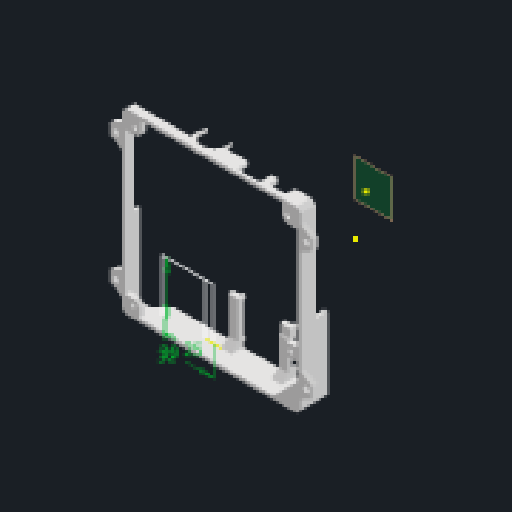
# Autodesk Inventor part: Buttom_part
Saved by Autodesk Inventor 2026.2 (Build 302298000, 298)
## iProperties
Created: 2026-04-25
Part Number: Buttom_part
Material: Generic
Document SubType Name: Modeling
Designer: Malthe Sennels
Density: 1 g/cm^3
Appearance: Default
Author: Malthe Sennels
Autodesk Inventor part; units mm, degrees
ref_plane "YZ Plane" through (0, 0, 0) normal (1, 0, 0) x (0, 1, 0)
ref_plane "XZ Plane" through (0, 0, 0) normal (0, 1, 0) x (-1, 0, 0)
ref_plane "XY Plane" through (0, 0, 0) normal (0, 0, 1) x (1, 0, 0)
sketch "Sketch1" plane through (0, 0, 0) normal (0, 0, 1) x (1, 0, 0)
  line L0 (-32, -107.75) -> (-32, -22.5) construction
  line L1 (-33, -21.5) -> (-131, -21.5) construction
  line L2 (-32, -22.5) -> (-33, -21.5) construction
  line L3 (-45.75, -121.5) -> (-32, -107.75) construction
  line L4 (-131, -121.5) -> (-45.75, -121.5) construction
  line L5 (-132, -120.5) -> (-131, -121.5) construction
  line L6 (-132, -22.5) -> (-132, -120.5) construction
  line L7 (-131, -21.5) -> (-132, -22.5) projected
  line L8 (-31.6, -22.3343) -> (-31.6, -107.9157)
  line L9 (-31.6, -107.9157) -> (-45.5843, -121.9)
  line L10 (-45.5843, -121.9) -> (-131.1657, -121.9)
  line L11 (-131.1657, -121.9) -> (-132.4, -120.6657)
  line L12 (-132.4, -120.6657) -> (-132.4, -22.3343)
  line L13 (-132.4, -22.3343) -> (-131.1657, -21.1)
  line L14 (-131.1657, -21.1) -> (-32.8343, -21.1)
  line L15 (-32.8343, -21.1) -> (-31.6, -22.3343)
  circle A0 centre (-37, -26.5) radius 1.25 projected
  circle A1 centre (-37, -26.5) radius 3.75
  line L16 (-40.75, -26.5) -> (-40.75, -21.1)
  line L17 (-37, -30.25) -> (-31.6, -30.25)
  circle A2 centre (-126.8952, -26.4793) radius 1.25 projected
  circle A3 centre (-126.8952, -26.4793) radius 3.75
  line L18 (-123.1452, -26.4793) -> (-123.1452, -21.1)
  line L19 (-126.8952, -30.2293) -> (-132.4, -30.2293)
  circle A4 centre (-127.9242, -117.4242) radius 1.25 projected
  circle A5 centre (-127.9242, -117.4242) radius 3.75
  line L20 (-124.1742, -117.4242) -> (-124.1742, -121.9)
  line L21 (-127.9242, -113.6742) -> (-132.4, -113.6742)
  circle A6 centre (-35.375, -94.25) radius 1.25 projected
  circle A7 centre (-35.375, -94.25) radius 3.75
  line L22 (-35.375, -98) -> (-31.6, -98)
  line L23 (-35.375, -90.5) -> (-31.6, -90.5)
  line L24 (-29.6, -108.7441) -> (-29.6, -21.5059)
  line L25 (-29.6, -21.5059) -> (-32.0059, -19.1)
  line L26 (-32.0059, -19.1) -> (-131.9941, -19.1)
  line L27 (-131.9941, -19.1) -> (-134.4, -21.5059)
  line L28 (-134.4, -21.5059) -> (-134.4, -121.4941)
  line L29 (-134.4, -121.4941) -> (-131.9941, -123.9)
  line L30 (-131.9941, -123.9) -> (-44.7559, -123.9)
  line L31 (-44.7559, -123.9) -> (-29.6, -108.7441)
  line L32 (-29.6, -108.7441) -> (-29.6, -121.4941)
  line L33 (-32.0059, -123.9) -> (-44.7559, -123.9)
  line L34 (-29.6, -121.4941) -> (-32.0059, -123.9)
  point P0 (0, 0)
  point P1 (-29.6, -123.9)
  dimension "d0" = 0.4
  dimension "d1" = 7.5
  dimension "d2" = 7.5
  dimension "d3" = 7.5
  dimension "d4" = 7.5
  dimension "d5" = 2
  dimension "d26" = 2.4059
  dimension "d27" = 2.4059
  dimension "d28" = 2.4059
  constraints: 54 end point, 11 point on line, 8 perpendicular, 8 point on circle, 8 tangent, 4 centre point, 4 coincident, 1 vertical, 14 other
  measures "d0" distance between parallel lines of L0 L8
  measures "d1" diameter of A1
  measures "d2" diameter of A3
  measures "d3" diameter of A5
  measures "d4" diameter of A7
  measures "d5" distance between parallel lines of L8 L24
  measures "d26" horizontal distance of L28.end L29.end
  measures "d27" distance of L32.end point (-29.6, -123.9)
  measures "d28" distance of L33.start point (-29.6, -123.9)
extrude "Extrusion1" add sketch "Sketch1" along normal blind 3 contours L8 L17 A1 L16 L14 L15 | L8 L22 A7 L23 | A1 | A7 | L18 A3 L19 L12 L13 L14 | A3 | L10 L11 L12 L21 A5 L20 | A5 | L31 L30 L29 L28 L27 L26 L25 L24 | L32 L34 L33 L31
sketch "Sketch3" plane through (0, 0, 0) normal (0, 0, -1) x (-1, 0, 0)
  line L0 (29.6, -21.5059) -> (32.0059, -19.1) projected
  line L1 (134.4, -121.4941) -> (131.9941, -123.9) projected
  line L2 (134.4, -21.5059) -> (134.4, -121.4941) projected
  line L3 (131.9941, -19.1) -> (134.4, -21.5059) projected
  line L4 (32.0059, -19.1) -> (131.9941, -19.1) projected
  circle A0 centre (35.375, -94.25) radius 1.25 projected
  circle A1 centre (127.9242, -117.4242) radius 1.25 projected
  circle A2 centre (37, -26.5) radius 1.25 projected
  circle A3 centre (126.8952, -26.4793) radius 1.25 projected
  arc A4 (123.1452, -26.4793) -> (126.8952, -30.2293) centre (126.8952, -26.4793) ccw projected
  line L5 (132.4, -30.2293) -> (126.8952, -30.2293) projected
  line L6 (132.4, -113.6742) -> (132.4, -30.2293) projected
  line L7 (127.9242, -113.6742) -> (132.4, -113.6742) projected
  arc A5 (127.9242, -113.6742) -> (124.1742, -117.4242) centre (127.9242, -117.4242) ccw projected
  line L8 (124.1742, -121.9) -> (124.1742, -117.4242) projected
  line L9 (45.5843, -121.9) -> (124.1742, -121.9) projected
  line L10 (31.6, -107.9157) -> (45.5843, -121.9) projected
  line L11 (31.6, -98) -> (31.6, -107.9157) projected
  line L12 (35.375, -98) -> (31.6, -98) projected
  arc A6 (35.375, -98) -> (35.375, -90.5) centre (35.375, -94.25) ccw projected
  line L13 (31.6, -90.5) -> (35.375, -90.5) projected
  line L14 (31.6, -30.25) -> (31.6, -90.5) projected
  line L15 (37, -30.25) -> (31.6, -30.25) projected
  arc A7 (37, -30.25) -> (40.75, -26.5) centre (37, -26.5) ccw projected
  line L16 (40.75, -21.1) -> (40.75, -26.5) projected
  line L17 (123.1452, -21.1) -> (40.75, -21.1) projected
  line L18 (123.1452, -26.4793) -> (123.1452, -21.1) projected
  line L19 (31.6, -22.3343) -> (32.8343, -21.1)
  line L20 (32.8343, -21.1) -> (131.1657, -21.1)
  line L21 (131.1657, -21.1) -> (132.4, -22.3343)
  line L22 (132.4, -22.3343) -> (132.4, -120.6657)
  line L23 (132.4, -120.6657) -> (131.1657, -121.9)
  line L24 (131.1657, -121.9) -> (45.5843, -121.9)
  line L25 (45.5843, -121.9) -> (31.6, -107.9157)
  line L26 (31.6, -107.9157) -> (31.6, -22.3343)
  line L27 (29.6, -121.4941) -> (29.6, -21.5059) projected
  line L28 (32.0059, -123.9) -> (29.6, -121.4941) projected
  line L29 (131.9941, -123.9) -> (32.0059, -123.9) projected
  point P0 (0, 0)
  point P1 (132.4, -41.5929)
  constraints: 16 end point, 4 other
extrude "Extrusion2" add sketch "Sketch3" along normal blind 6 contours L0 L4 L3 L2 L1 L29 L28 L27
sketch "Sketch4" plane through (-131.9941, -19.1, 3) normal (0, 1, 0) x (1, 0, 0)
  line L0 (65.2616, 3) -> (65.2616, 4.5558) projected
  line L1 (74.5016, 3) -> (74.5016, 4.5558) projected
  line L2 (98.9941, 3) -> (0.9941, 3) projected
  line L3 (99.1598, 9) -> (0.8284, 9) projected
  line L4 (63.2616, 8) -> (63.2616, 3)
  line L5 (64.2616, 2) -> (75.5016, 2)
  line L6 (76.5016, 3) -> (76.5016, 8)
  arc A0 (63.2616, 3) -> (64.2616, 2) centre (64.2616, 3) ccw
  arc A1 (75.5016, 2) -> (76.5016, 3) centre (75.5016, 3) ccw
  line L7 (62.2616, 9) -> (61.3217, 9)
  line L8 (77.5016, 9) -> (78.7059, 9)
  line L9 (63.2616, 9) -> (76.5016, 9)
  arc A2 (63.2616, 8) -> (62.2616, 9) centre (62.2616, 8) ccw
  arc A3 (77.5016, 9) -> (76.5016, 8) centre (77.5016, 8) ccw
  line L10 (87.1737, 4.5558) -> (88.7737, 4.5558) projected
  line L11 (82.0937, 4.5558) -> (83.6937, 4.5558) projected
  line L12 (80.5937, 8) -> (80.5937, 4.5558)
  line L13 (81.5937, 3.5558) -> (89.2737, 3.5558)
  line L14 (90.2737, 4.5558) -> (90.2737, 8)
  arc A4 (80.5937, 4.5558) -> (81.5937, 3.5558) centre (81.5937, 4.5558) ccw
  arc A5 (89.2737, 3.5558) -> (90.2737, 4.5558) centre (89.2737, 4.5558) ccw
  line L15 (77.5016, 9) -> (79.5937, 9)
  arc A6 (80.5937, 8) -> (79.5937, 9) centre (79.5937, 8) ccw
  line L16 (102.3941, 9) -> (102.3941, 0) projected
  line L17 (91.2737, 9) -> (102.3941, 9)
  arc A7 (91.2737, 9) -> (90.2737, 8) centre (91.2737, 8) ccw
  point P0 (131.9941, 3)
  point P1 (80.5937, 9)
  point P2 (90.2737, 9)
  dimension "d11" = 2
  dimension "d12" = 2
  dimension "d13" = 1
  dimension "d14" = 1
  dimension "d15" = 1
  dimension "d32" = 1.5
  dimension "d33" = 1.5
  dimension "d34" = 1
  dimension "d35" = 1
  dimension "d36" = 1
  dimension "d37" = 1
  constraints: 22 end point, 16 point on circle, 16 tangent, 14 point on line, 8 centre point, 4 perpendicular, 3 equal radius, 2 horizontal, 2 vertical, 1 collinear
  measures "d11" distance between parallel lines of L6 L1
  measures "d12" distance between parallel lines of L4 L0
  measures "d13" distance between parallel lines of L2 L5
  measures "d14" radius of A0
  measures "d15" radius of A2
  measures "d32" distance from line of L12 L11.start
  measures "d33" distance from line of L14 L10.end
  measures "d34" distance between parallel lines of L11 L13
  measures "d35" radius of A4
  measures "d36" radius of A6
  measures "d37" radius of A7
extrude "Extrusion3" cut sketch "Sketch4" against normal up to surface (2 mm away)
sketch "Sketch5" plane through (0, 0, 3) normal (0, 0, 1) x (1, 0, 0)
  circle A0 centre (-26.1, -34.1) radius 1.75
  line L0 (-29.6, -108.7441) -> (-29.6, -21.5059) projected
  line L1 (-29.6, -27.0585) -> (-22.6, -31.1)
  line L2 (-22.6, -31.1) -> (-22.6, -37.1)
  line L3 (-22.6, -37.1) -> (-29.6, -41.1415)
  line L4 (-22.6, -34.1) -> (-29.6, -34.1) construction
  line L5 (-32.0059, -19.1) -> (-131.9941, -19.1) projected
  line L6 (-29.6, -21.5059) -> (-29.6, -121.4941)
  line L7 (-29.6, -71.5) -> (-134.4, -71.5)
  line L8 (-134.4, -21.5059) -> (-134.4, -121.4941) projected
  circle A1 centre (-26.1, -108.9) radius 1.75
  line L9 (-29.6, -115.9415) -> (-22.6, -111.9)
  line L10 (-22.6, -111.9) -> (-22.6, -105.9)
  line L11 (-22.6, -105.9) -> (-29.6, -101.8585)
  line L12 (-22.6, -108.9) -> (-29.6, -108.9) construction
  line L13 (-82, -19.1) -> (-82, -123.9)
  line L14 (-131.9941, -123.9) -> (-32.0059, -123.9) projected
  circle A2 centre (-137.9, -34.1) radius 1.75
  line L15 (-134.4, -27.0585) -> (-141.4, -31.1)
  line L16 (-141.4, -31.1) -> (-141.4, -37.1)
  line L17 (-141.4, -37.1) -> (-134.4, -41.1415)
  line L18 (-141.4, -34.1) -> (-134.4, -34.1) construction
  line L19 (-134.4, -115.9415) -> (-141.4, -111.9)
  line L20 (-141.4, -108.9) -> (-134.4, -108.9) construction
  circle A3 centre (-137.9, -108.9) radius 1.75
  line L21 (-141.4, -105.9) -> (-134.4, -101.8585)
  line L22 (-141.4, -111.9) -> (-141.4, -105.9)
  point P0 (0, 0)
  point P1 (-134.4, -108.7441)
  dimension "d19" = 120
  dimension "d20" = 120
  dimension "d21" = 3.5
  dimension "d22" = 3.5
  dimension "d23" = 7
  dimension "d24" = 3
  dimension "d25" = 15
  constraints: 38 end point, 22 symmetric about line, 9 midpoint, 4 centre point, 3 point on line, 1 parallel, 1 perpendicular, 3 other
  measures "d19" angle of L2 L3
  measures "d20" angle of L2 L1
  measures "d21" distance from line of L0 A0.centre
  measures "d22" diameter of A0
  measures "d23" distance between parallel lines of L0 L2
  measures "d24" distance from line of L1.end L4
  measures "d25" distance between parallel lines of L5 L4
extrude "Extrusion4" add sketch "Sketch5" against normal blind 3
sketch "Sketch6" plane through (0, 0, -6) normal (0, 0, -1) x (-1, 0, 0)
  point P0 (0, 0)
sketch "Sketch7" plane through (-131.9941, -19.1, 3) normal (0, 1, 0) x (1, 0, 0)
  circle A0 centre (40.9941, 10.95) radius 3.9 projected
  circle A1 centre (40.9941, 10.95) radius 2.9
  line L0 (0, 9) -> (62.2616, 9) projected
  line L1 (49.2757, 9) -> (48.3941, 14)
  line L2 (48.3941, 14) -> (43.8941, 14)
  line L3 (43.8941, 14) -> (43.8941, 10.95)
  line L4 (40.9941, 7.05) -> (40.9941, 14.85)
  line L5 (32.7125, 9) -> (33.5941, 14)
  line L6 (33.5941, 14) -> (38.0941, 14)
  line L7 (38.0941, 14) -> (38.0941, 10.95)
  point P0 (131.9941, 3)
  point P1 (43.1406, 9)
  point P2 (32.7125, 9)
  point P3 (38.8476, 9)
  dimension "d38" = 5.8
  dimension "d39" = 80
  dimension "d40" = 5
  dimension "d41" = 4.5
  constraints: 14 end point, 4 symmetric about line, 3 vertical, 2 point on circle, 1 coincident, 1 parallel, 1 perpendicular, 1 point on line, 3 other
  measures "d39" angle of L0 L1
  measures "d40" distance between parallel lines of L0 L2
  measures "d41" distance of L2.end L1.end
extrude "Extrusion5" add sketch "Sketch7" against normal up to surface (2 mm away) contours A0 L0 A1 L3 | A0 L3 L2 L1 L0 | L7 A1 L0 A0 | A0 L0 L5 L6 L7
sketch "Sketch8" plane through (-131.9941, -19.1, 3) normal (0, 1, 0) x (1, 0, 0)
  arc A0 (43.1406, 9) -> (43.8941, 10.95) centre (40.9941, 10.95) ccw projected
  circle A1 centre (40.9941, 10.95) radius 2.9
  point P0 (131.9941, 3)
  point P1 (43.1406, 9)
  constraints: 1 coincident, 3 other
extrude "Extrusion6" cut sketch "Sketch8" against normal up to surface (2 mm away)
sketch "Sketch9" plane through (0, 0, -6) normal (0, 0, -1) x (-1, 0, 0)
  line L0 (94.6, -132.1582) -> (23.2926, -132.1582)
  line L1 (23.2926, -132.1582) -> (23.2926, -78.9)
  line L2 (23.2926, -78.9) -> (94.6, -78.9)
  line L3 (94.6, -78.9) -> (94.6, -132.1582)
  line L4 (99.2816, -19.1) -> (99.2816, -21.1) projected
  line L5 (99.2816, -21.1) -> (131.1657, -21.1) projected
  line L6 (131.1657, -21.1) -> (132.4, -22.3343) projected
  line L7 (132.4, -22.3343) -> (132.4, -120.6657) projected
  line L8 (132.4, -120.6657) -> (131.1657, -121.9) projected
  line L9 (131.1657, -121.9) -> (45.5843, -121.9) projected
  line L10 (45.5843, -121.9) -> (31.6, -107.9157) projected
  line L11 (31.6, -107.9157) -> (31.6, -22.3343) projected
  line L12 (31.6, -22.3343) -> (32.8343, -21.1) projected
  line L13 (32.8343, -21.1) -> (40.7204, -21.1) projected
  line L14 (40.7204, -21.1) -> (40.7204, -19.1) projected
  line L15 (40.7204, -19.1) -> (32.0059, -19.1) projected
  line L16 (32.0059, -19.1) -> (29.6, -21.5059) projected
  line L17 (29.6, -21.5059) -> (29.6, -121.4941) projected
  line L18 (29.6, -121.4941) -> (32.0059, -123.9) projected
  line L19 (32.0059, -123.9) -> (131.9941, -123.9) projected
  line L20 (131.9941, -123.9) -> (134.4, -121.4941) projected
  line L21 (134.4, -121.4941) -> (134.4, -21.5059) projected
  line L22 (134.4, -21.5059) -> (131.9941, -19.1) projected
  line L23 (131.9941, -19.1) -> (99.2816, -19.1) projected
  line L24 (32.0059, -123.9) -> (131.9941, -123.9) projected
  line L25 (29.6, -21.5059) -> (29.6, -121.4941) projected
  point P0 (0, 0)
  point P1 (31.6, -78.9)
  point P2 (29.6, -78.9)
  point P3 (94.6, -123.9)
  point P4 (94.6, -121.9)
  dimension "d46" = 45
  dimension "d47" = 65
  constraints: 8 end point, 2 parallel, 1 horizontal, 1 perpendicular
  measures "d46" distance between parallel lines of L2 L24
  measures "d47" distance between parallel lines of L3 L25
extrude "Extrusion7" add sketch "Sketch9" along normal blind 7 contours L19 L18 L17 L2 L11 L10 L9 L3
sketch "Sketch10" plane through (0, 0, -13) normal (0, 0, -1) x (-1, 0, 0)
  line L0 (32.0059, -123.9) -> (94.6, -123.9) projected
  line L1 (54.6, -123.9) -> (48.6, -123.9)
  line L2 (48.6, -123.9) -> (48.6, -95.9)
  line L3 (48.6, -95.9) -> (54.6, -95.9)
  line L4 (54.6, -95.9) -> (54.6, -123.9)
  line L5 (85.08, -123.9) -> (79.08, -123.9)
  line L6 (79.08, -123.9) -> (79.08, -95.9)
  line L7 (79.08, -95.9) -> (85.08, -95.9)
  line L8 (85.08, -95.9) -> (85.08, -123.9)
  line L9 (82.08, -95.9) -> (82.08, -123.9)
  line L10 (51.6, -95.9) -> (51.6, -123.9)
  line L11 (29.6, -78.9) -> (29.6, -121.4941) projected
  point P0 (0, 0)
  dimension "d50" = 30.48
  dimension "d51" = 6
  dimension "d52" = 6
  dimension "d53" = 28
  dimension "d54" = 22
  constraints: 20 end point, 4 midpoint, 4 parallel, 3 point on line, 2 horizontal, 2 perpendicular
  measures "d50" distance between parallel lines of L10 L9
  measures "d51" distance between parallel lines of L2 L4
  measures "d52" distance between parallel lines of L8 L6
  measures "d53" distance between parallel lines of L0 L7
  measures "d54" distance between parallel lines of L11 L10
extrude "Extrusion8" add sketch "Sketch10" against normal blind 3
sketch "Sketch11" plane through (0, 0, -13) normal (0, 0, -1) x (-1, 0, 0)
  line L0 (79.08, -95.9) -> (85.08, -95.9) projected
  line L1 (82.08, -95.9) -> (82.08, -125.121) construction
  line L2 (54.6, -95.9) -> (48.6, -95.9) projected
  line L3 (51.6, -95.9) -> (51.6, -123.9) construction
  line L4 (32.0059, -123.9) -> (94.6, -123.9) projected
  circle A0 centre (82.08, -120.16) radius 1.4
  circle A1 centre (82.08, -98.9) radius 1.4
  line L5 (85.08, -95.9) -> (79.08, -95.9) projected
  line L6 (82.08, -120.16) -> (51.6, -120.16)
  line L7 (82.08, -98.9) -> (51.6, -98.9)
  circle A2 centre (51.6, -120.16) radius 1.4
  circle A3 centre (51.6, -98.9) radius 1.4
  point P0 (0, 0)
  dimension "d57" = 2.8
  dimension "d58" = 2.8
  dimension "d59" = 21.26
  dimension "d60" = 3
  dimension "d61" = 2.8
  dimension "d62" = 2.8
  constraints: 8 end point, 5 point on line, 4 centre point, 2 coincident, 2 midpoint, 2 perpendicular, 2 vertical
  measures "d57" diameter of A0
  measures "d58" diameter of A1
  measures "d59" distance of L7.start L6.start
  measures "d60" distance from line of L5 L7.start
  measures "d61" diameter of A2
  measures "d62" diameter of A3
extrude "Extrusion9" add sketch "Sketch11" along normal blind 3
sketch "Sketch12" plane through (-48.6, -121.9, -13) normal (1, 0, 0) x (0, 0, -1)
  line L0 (0, 20) -> (-2, 18)
  line L1 (-2, 18) -> (-2, 7)
  line L2 (-2, 7) -> (0, 5)
  line L3 (0, 0) -> (0, 26) projected
  line L4 (0, 0) -> (0, 26) projected
  line L5 (-7, -2) -> (0, -2) projected
  point P0 (-13, 121.9)
  point P1 (0, 13)
  point P2 (0, 20)
  dimension "d65" = 135
  dimension "d66" = 135
  dimension "d67" = 2
  dimension "d68" = 8
  dimension "d69" = 9
  constraints: 6 end point, 2 point on line, 1 midpoint, 1 parallel
  measures "d65" angle of L4 L0
  measures "d66" angle of L4 L2
  measures "d67" distance from line of point (0, 13) L1
  measures "d68" vertical distance of L3.end L0.end
  measures "d69" distance from line of L1.end L5
extrude "Extrusion10" cut sketch "Sketch12" against normal up to surface (6 mm away)
sketch "Sketch13" plane through (-48.6, -121.9, -10) normal (1, 0, 0) x (0, 0, -1)
  line L0 (3, 20) -> (1, 18) projected
  line L1 (1, 7) -> (3, 5) projected
  line L2 (1, 22.2426) -> (-1, 20.2426)
  line L3 (-1.1213, 4.8787) -> (0.8787, 2.8787)
  line L4 (-1, 20.2426) -> (-1, 0)
  line L5 (-4, 0) -> (3, 0) projected
  line L6 (3, 0) -> (3, 5) projected
  line L7 (0, 21.2426) -> (0, 0)
  point P0 (-10, 121.9)
  dimension "d72" = 3
  dimension "d73" = 3
  dimension "d74" = 4
  constraints: 8 end point, 3 point on line, 2 parallel, 2 perpendicular, 1 midpoint
  measures "d72" distance between parallel lines of L0 L2
  measures "d73" distance between parallel lines of L1 L3
  measures "d74" distance between parallel lines of L6 L4
extrude "Extrusion11" add sketch "Sketch13" against normal up to surface (6 mm away)
chamfer "Chamfer1" distance 4 angle 45 2 edges at (-82.08, -121.9, -10) (-51.6, -121.9, -9)
sketch "Sketch14" plane through (0, 0, -6) normal (0, 0, -1) x (-1, 0, 0)
  line L0 (94.6, -123.9) -> (131.9941, -123.9) projected
  line L1 (94.6, -123.9) -> (119.6, -123.9)
  line L2 (119.6, -123.9) -> (119.6, -91.9)
  line L3 (119.6, -91.9) -> (94.6, -91.9)
  line L4 (94.6, -91.9) -> (94.6, -123.9)
  line L5 (94.6, -121.9) -> (85.08, -121.9) projected
  line L6 (94.6, -91.9) -> (89.6, -91.9)
  line L7 (89.6, -91.9) -> (89.6, -121.9)
  line L8 (89.6, -121.9) -> (94.6, -121.9)
  line L9 (94.6, -121.9) -> (94.6, -91.9)
  point P0 (0, 0)
  dimension "d80" = 32
  dimension "d81" = 25
  dimension "d82" = 30
  constraints: 16 end point, 4 parallel, 2 horizontal, 2 perpendicular, 1 point on line
  measures "d80" distance between parallel lines of L0 L3
  measures "d81" distance between parallel lines of L4 L2
  measures "d82" distance between parallel lines of L2 L7
ref_plane "Work Plane1" through (0, 0, -10) normal (0, 0, -1) x (-1, 0, 0)
sketch "Sketch15" plane through (0, 0, -10) normal (0, 0, -1) x (-1, 0, 0)
  line L0 (94.6, -123.9) -> (94.6, -121.9) projected
  line L1 (94.6, -123.9) -> (119.6, -123.9) projected
  line L2 (119.6, -123.9) -> (119.6, -91.9) projected
  line L3 (119.6, -121.9) -> (94.6, -121.9)
  point P0 (0, 0)
  constraints: 2 end point, 1 horizontal, 1 point on line
extrude "Extrusion13" add sketch "Sketch15" along normal up to surface (3 mm away)
sketch "Sketch16" plane through (0, 0, -6) normal (0, 0, -1) x (-1, 0, 0)
  line L0 (145.0581, -74.1) -> (99.4, -74.1)
  line L1 (99.4, -74.1) -> (99.4, -16.8745)
  line L2 (99.4, -16.8745) -> (145.0581, -16.8745)
  line L3 (145.0581, -16.8745) -> (145.0581, -74.1)
  line L4 (94.6, -123.9) -> (131.9941, -123.9) projected
  line L5 (131.9941, -123.9) -> (134.4, -121.4941) projected
  line L6 (134.4, -121.4941) -> (134.4, -21.5059) projected
  line L7 (134.4, -21.5059) -> (131.9941, -19.1) projected
  line L8 (131.9941, -19.1) -> (99.2816, -19.1) projected
  line L9 (99.2816, -19.1) -> (99.2816, -21.1) projected
  line L10 (99.2816, -21.1) -> (131.1657, -21.1) projected
  line L11 (131.1657, -21.1) -> (132.4, -22.3343) projected
  line L12 (132.4, -22.3343) -> (132.4, -120.6657) projected
  line L13 (132.4, -120.6657) -> (131.1657, -121.9) projected
  line L14 (131.1657, -121.9) -> (94.6, -121.9) projected
  line L15 (131.9941, -19.1) -> (99.2816, -19.1) projected
  line L16 (134.4, -121.4941) -> (134.4, -21.5059) projected
  line L17 (94.6, -121.9) -> (94.6, -123.9) projected
  point P0 (0, 0)
  point P1 (132.4, -74.1)
  point P2 (134.4, -74.1)
  dimension "d92" = 55
  dimension "d93" = 35
  constraints: 8 end point, 2 parallel, 1 horizontal, 1 perpendicular
  measures "d92" distance between parallel lines of L0 L15
  measures "d93" distance between parallel lines of L16 L1
extrude "Extrusion14" cut sketch "Sketch16" against normal blind 4 contours L0 L12 L11 L10 L1 L8 L7 L6 | L1 L10 L9 L8
sketch "Sketch17" plane through (0, 0, -6) normal (0, 0, -1) x (-1, 0, 0)
  point P0 (0, 0)
sketch "Sketch18" plane through (-124.1742, -121.9, 3) normal (0, 1, 0) x (1, 0, 0)
  line L0 (4.5742, 13) -> (4.5742, 16) projected
  line L1 (4.5742, 16) -> (-2.4258, 9)
  line L2 (-6.9915, 9) -> (29.5742, 9) projected
  line L3 (4.5742, 16) -> (14.4737, 16) construction
  line L4 (4.5742, 13) -> (29.5742, 13) projected
  line L5 (4.5742, 9) -> (29.5742, 9) projected
  line L6 (29.5742, 9) -> (29.5742, 13) projected
  point P0 (124.1742, 3)
  dimension "d94" = 135
  constraints: 4 end point, 1 equal length, 1 horizontal, 1 point on line
  measures "d94" angle of L1 L3
extrude "Extrusion15" add sketch "Sketch18" against normal up to surface (2 mm away)
sketch "Sketch19" plane through (-123.1452, -21.1, 3) normal (0, -1, 0) x (1, 0, 0)
  point P0 (123.1452, -3)
sketch "Sketch22" plane through (-131.9941, -19.1, 3) normal (0, 1, 0) x (1, 0, 0)
  spline S0 degree 8 number of poles 65
  spline S1 degree 8 number of poles 65
  spline S2 degree 6 poles (40.9941, 14.0948) (40.6733, 14.0874) (40.3534, 14.0408) (40.0407, 13.955) (39.7411, 13.8313) (39.4603, 13.6721) (38.9467, 13.2906) (38.7138, 13.0683) (38.5096, 12.818) (38.3383, 12.5444) (38.2031, 12.2526) (38.0129, 11.658) (37.9547, 11.3559) (37.9333, 11.0481) (37.9493, 10.7401) (38.0022, 10.4375) (38.1787, 9.8546) (38.3021, 9.5741) (38.4593, 9.31) (38.6474, 9.0671) (38.863, 8.8499) (39.3323, 8.4805) (39.5845, 8.3262) (39.8542, 8.2028) (40.1365, 8.1125) (40.4265, 8.057) (41.0045, 8.0166) (41.2925, 8.0302) (41.5777, 8.0778) (41.8551, 8.1588) (42.1199, 8.2717) (42.6099, 8.553) (42.8358, 8.7202) (43.0413, 8.9131) (43.2227, 9.1287) (43.377, 9.3632) (43.5572, 9.7225) (43.6068, 9.8358) (43.6504, 9.9515) (43.6879, 10.0694) (43.7192, 10.1889) (43.7441, 10.3097) knots 0 0 0 0 0 0 0 0.133235 0.133235 0.133235 0.133235 0.133235 0.266244 0.266244 0.266244 0.266244 0.266244 0.393711 0.393711 0.393711 0.393711 0.393711 0.520997 0.520997 0.520997 0.520997 0.520997 0.644189 0.644189 0.644189 0.644189 0.644189 0.764658 0.764658 0.764658 0.764658 0.764658 0.882458 0.882458 0.882458 0.882458 0.882458 0.934692 0.934692 0.934692 0.934692 0.934692 0.934692 0.934692
  circle A0 centre (40.9941, 10.9699) radius 7.5
  point P0 (131.9941, 3)
  dimension "d106" = 15
  constraints: 1 centre point, 10 other
  measures "d106" diameter of A0
extrude "Extrusion18" cut sketch "Sketch22" against normal up to surface (2 mm away)
sketch "Sketch23" plane through (-131.9941, -19.1, 3) normal (0, 1, 0) x (1, 0, 0)
  line L0 (49.2757, 9) -> (48.3941, 14) projected
  line L1 (48.3941, 14) -> (55.7757, 14)
  line L2 (55.7757, 14) -> (60.7757, 9)
  line L3 (49.2757, 9) -> (62.2616, 9) projected
  point P0 (131.9941, 3)
  dimension "d109" = 45
  dimension "d110" = 6.5
  constraints: 4 end point, 1 parallel, 1 point on line
  measures "d109" angle of L3 L2
  measures "d110" horizontal distance of L0.start L1.end
extrude "Extrusion19" add sketch "Sketch23" against normal up to surface (2 mm away)
sketch "Sketch24" plane through (-131.9941, -19.1, 3) normal (0, 1, 0) x (1, 0, 0)
  arc A0 (34.1335, 14) -> (47.8548, 14) centre (40.9941, 10.9699) ccw projected
  line L0 (34.1335, 14) -> (33.5941, 14) projected
  line L1 (33.5941, 14) -> (32.7125, 9) projected
  line L2 (32.7125, 9) -> (32.7125, 5) projected
  line L3 (32.7125, 5) -> (0, 5) projected
  line L4 (0, 5) -> (0, 0) projected
  line L5 (99.9882, 0) -> (0, 0) projected
  line L6 (99.9882, 9) -> (99.9882, 0) projected
  line L7 (91.2737, 9) -> (99.9882, 9) projected
  arc A1 (91.2737, 9) -> (90.2737, 8) centre (91.2737, 8) ccw projected
  line L8 (90.2737, 8) -> (90.2737, 4.5558) projected
  arc A2 (89.2737, 3.5558) -> (90.2737, 4.5558) centre (89.2737, 4.5558) ccw projected
  line L9 (89.2737, 3.5558) -> (81.5937, 3.5558) projected
  arc A3 (80.5937, 4.5558) -> (81.5937, 3.5558) centre (81.5937, 4.5558) ccw projected
  line L10 (80.5937, 4.5558) -> (80.5937, 8) projected
  arc A4 (80.5937, 8) -> (79.5937, 9) centre (79.5937, 8) ccw projected
  line L11 (77.5016, 9) -> (79.5937, 9) projected
  arc A5 (77.5016, 9) -> (76.5016, 8) centre (77.5016, 8) ccw projected
  line L12 (76.5016, 8) -> (76.5016, 3) projected
  arc A6 (75.5016, 2) -> (76.5016, 3) centre (75.5016, 3) ccw projected
  line L13 (75.5016, 2) -> (64.2616, 2) projected
  arc A7 (63.2616, 3) -> (64.2616, 2) centre (64.2616, 3) ccw projected
  line L14 (63.2616, 3) -> (63.2616, 8) projected
  arc A8 (63.2616, 8) -> (62.2616, 9) centre (62.2616, 8) ccw projected
  line L15 (60.7757, 9) -> (62.2616, 9) projected
  line L16 (60.7757, 9) -> (55.7757, 14) projected
  line L17 (55.7757, 14) -> (47.8548, 14) projected
  line L18 (32.7125, 5) -> (36.4543, 5)
  point P0 (131.9941, 3)
  constraints: 2 end point, 1 horizontal, 1 point on circle
extrude "Extrusion20" cut sketch "Sketch24" against normal up to surface (2 mm away) contours A0 L18 L2 L1 L0
equation "\"d27\" = d26"
equation "\"d28\" = d27"
equation "\"d19\" = d20"
equation "\"d58\" = d57"
equation "\"d61\" = d57"
equation "\"d62\" = d57"
body "Solid1"
